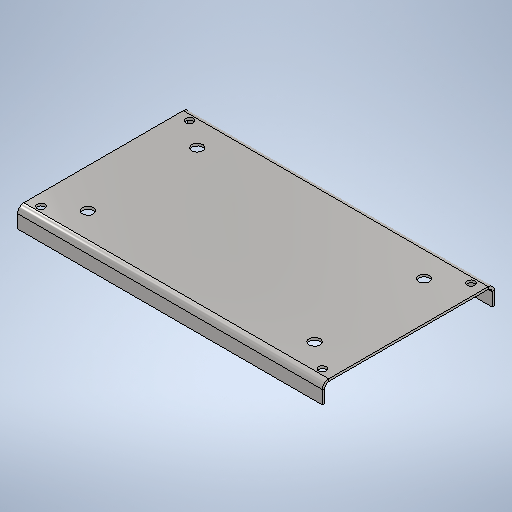
# Autodesk Inventor part: AIRPUMP plate
Saved by Autodesk Inventor 2025 (Build 290162010, 162A)
## iProperties
Created: 2024-12-06
Part Number: AIRPUMP plate
Material: Stainless Steel
Document SubType Name: Sheet Metal
Designer: pokla
Density: 8 g/cm^3
Sheet Metal Rule: AISI304 3mm Die 32
Appearance: Semi-Polished
Mass: 2396.5 g
Surface Area: 2045.03 cm^2
Volume: 299.562 cm^3
Flat Pattern Width: 25.7855 cm
Flat Pattern Length: 39 cm
Flat Pattern Area: 1005.63 cm^2
Sheet Metal Width: 257,855 mm
Sheet Metal Length: 390,000 mm
Sheet Metal Area: 100563,398 mm^2
Author: pokla
Autodesk Inventor part; units mm, degrees
ref_plane "YZ Plane" through (0, 0, 0) normal (1, 0, 0) x (0, 1, 0)
ref_plane "XZ Plane" through (0, 0, 0) normal (0, 1, 0) x (-1, 0, 0)
ref_plane "XY Plane" through (0, 0, 0) normal (0, 0, 1) x (1, 0, 0)
sketch "Sketch1" plane through (0, 0, 0) normal (0, 0, 1) x (1, 0, 0)
  line L0 (-195, 110) -> (195, 110)
  line L1 (195, 110) -> (195, -110)
  line L2 (195, -110) -> (-195, -110)
  line L3 (-195, -110) -> (-195, 110)
  line L4 (-195, 110) -> (195, -110) construction
  point P0 (0, 0)
  point P1 (0, 0)
  dimension "d0" = 390
  dimension "d1" = 220
  measures "d0" distance of L0.start L0.end
  measures "d1" distance of L2.end L0.start
extrude "Plate1" add sketch "Sketch1" against normal blind 3
sketch "Sketch2" plane through (0, 0, 0) normal (0, 0, 1) x (1, 0, 0)
  line L0 (-145, 70) -> (145, 70) construction
  line L1 (145, 70) -> (145, -70) construction
  line L2 (145, -70) -> (-145, -70) construction
  line L3 (-145, -70) -> (-145, 70) construction
  line L4 (195, -110) -> (195, 110) projected
  point P0 (0, 0)
  point P1 (-145, 0)
  point P2 (0, 70)
  dimension "d3" = 290
  dimension "d4" = 140
  constraints: 8 end point, 4 coincident, 2 midpoint, 2 parallel, 1 horizontal, 1 horizontal alignment, 1 perpendicular, 1 vertical alignment
  measures "d3" distance of L0.start L0.end
  measures "d4" distance of L0.end L1.end
hole "Hole1" at (-145, 70, 0) at (145, 70, 0) at (-145, -70, 0) at (145, -70, 0) direction (0, 0, -1) diameter 14 end through all
sketch "Sketch3" plane through (0, 0, 0) normal (0, 0, 1) x (1, 0, 0)
  line L0 (-180, 95) -> (180, 95) construction
  line L1 (180, 95) -> (180, -95) construction
  line L2 (180, -95) -> (-180, -95) construction
  line L3 (-180, -95) -> (-180, 95) construction
  line L4 (-180, 95) -> (180, -95) construction
  point P0 (0, 0)
  point P1 (0, 0)
  dimension "d14" = 190
  dimension "d15" = 360
  constraints: 10 end point, 5 coincident, 2 parallel, 1 horizontal, 1 midpoint, 1 perpendicular
  measures "d14" distance of L2.end L0.start
  measures "d15" distance of L0.start L0.end
hole "Hole2" at (-180, 95, 0) at (180, 95, 0) at (180, -95, 0) at (-180, -95, 0) direction (0, 0, -1) diameter 10 end through all
sketch "Sketch4" plane through (-195, -107, 0) normal (0, -1, 0) x (1, 0, 0)
  line L0 (390, 0) -> (0, 0)
  line L1 (0, 0) -> (0, -25)
  line L2 (0, -25) -> (390, -25)
  line L3 (390, -25) -> (390, 0)
  constraints: 6 end point, 1 horizontal, 1 perpendicular, 1 vertical
edge flange "Flange1" height 25 angle 90 thickness 3 bend radius 5 thickness toward (0, -1, 0) relief round relief width 3 relief depth 1.5 corner gap 5 corner form 0 edges at (0, -110, -3) (0, 110, -3) wall of the first edge with corners at (195, -107, 0) (-195, -107, 0) (-195, -107, -25) (195, -107, -25)
bend "Bend1"
corner "Corner1"
equation "\"d11\" = Thickness"
equation "\"d2\" = Thickness"
equation "\"d23\" = BendReliefWidth"
equation "\"d24\" = BendReliefDepth"
equation "\"d25\" = MinimumRemnant"
equation "\"d26\" = TransitionRadius"
equation "\"d29\" = BendRadius"
equation "\"d30\" = CornerReliefSize"
equation "\"d31\" = GapSize"
equation "\"d32\" = JacobiRadiusSize"
equation "\"BendReliefWidth\" = Thickness"
equation "\"BendReliefDepth\" = 0.5 * Thickness"
equation "\"CornerReliefSize\" = 4 * Thickness"
equation "\"MinimumRemnant\" = 2 * Thickness"
equation "\"TransitionRadius\" = BendRadius"
equation "\"JacobiRadiusSize\" = BendRadius"
equation "\"GapSize\" = Thickness"
equation "\"Thickness\" = 3"
equation "\"BendRadius\" = 5"
body "Solid1"
